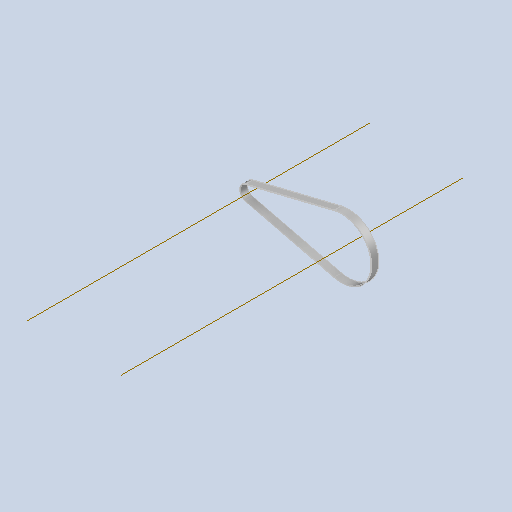
# Autodesk Inventor part: 歯付きベルト
Saved by Autodesk Inventor 2025 (Build 290162000, 162)
## iProperties
Created: 2024-06-24
Part Number: 歯付きベルト
Material: Rubber
Document SubType Name: Modeling
Designer: 8326d
Density: 1 g/cm^3
Appearance: Rubber - Black - Version 1.1
CustomPartVersion: 1
Author: 8326d
Autodesk Inventor part; units mm, degrees
ref_plane "YZ Plane" through (0, 0, 0) normal (1, 0, 0) x (0, 1, 0)
ref_plane "XZ Plane" through (0, 0, 0) normal (0, 1, 0) x (-1, 0, 0)
ref_plane "XY Plane" through (0, 0, 0) normal (0, 0, 1) x (1, 0, 0)
sketch "スケッチ パス" plane through (0, 0, 0) normal (0, 0, 1) x (1, 0, 0)
  arc A0 (-101.515735, 6.183124) -> (-101.515735, -6.183124) centre (-100, 0) ccw
  arc A1 (-25.847475, -24.732495) -> (-25.847475, 24.732495) centre (-19.784533, 0) ccw
  line L0 (-25.847475, -24.732495) -> (-101.515735, -6.183124)
  line L1 (-101.515735, 6.183124) -> (-25.847475, 24.732495)
  constraints: 4 end point, 4 point on circle, 2 centre point
ref_plane "断面平面" through (-101.515735, -6.183124, 0) normal (0.9712428, -0.2380912, 0) x (0, 0, 1)
ref_plane "作業平面2" through (-100, 0, 0) normal (-1, 0, 0) x (0, 0, 1)
ref_plane "作業平面3" through (-19.784533, 0, 0) normal (-0.9807853, -0.1950902, 0) x (0, 0, 1)
sketch "断面" plane through (-101.515735, -6.183124, 0) normal (0.9712428, -0.2380912, 0) x (0, 0, 1)
  line L0 (-3, 0.3) -> (3, 0.3)
  line L1 (3, 0.3) -> (3, -0.3)
  line L2 (3, -0.3) -> (-3, -0.3)
  line L3 (-3, -0.3) -> (-3, 0.3)
  line L4 (-3, 0) -> (3, 0) construction
  point P0 (0, 0)
  point P1 (0, 0)
  dimension "d0" = 6
  dimension "d4" = 0.3
  dimension "d5" = 0.3
  constraints: 10 end point, 3 midpoint, 2 parallel, 1 coincident, 1 horizontal, 1 perpendicular, 1 other
  measures "d0" distance between parallel lines of L1 L3
  measures "d4" distance between parallel lines of L2 L4
  measures "d5" distance between parallel lines of L4 L0
sweep "ベルト" add profiles "断面" path "スケッチ パス" path curves L1 A1 L0 A0
equation "\"d0\" = da_B"
equation "\"d4\" = da_a"
equation "\"d5\" = da_a2"
equation "\"da_B\" = 6"
equation "\"da_pb\" = 2.5"
equation "\"da_L\" = 265"
equation "\"da_a\" = 0.3"
equation "\"da_S\" = 1.5"
equation "\"da_Beta\" = 20deg"
equation "\"da_Ht\" = 0.7"
equation "\"da_H\" = 1.3"
equation "\"da_a2\" = 0.3"
body "Solid1"
